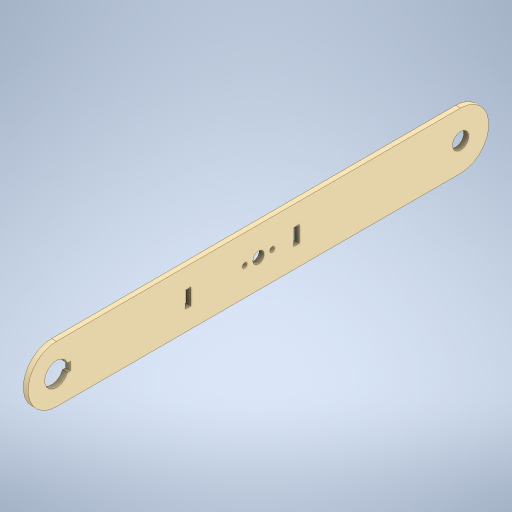
# Autodesk Inventor part: brazo2
Saved by Autodesk Inventor 2024.3 (Build 283343000, 343)
## iProperties
Created: 2024-05-14
Part Number: brazo2
Material: PMMA Plastic
Document SubType Name: Modeling
Designer: USUARIO
Density: 1.188 g/cm^3
Appearance: Beige
Mass: 33.3029 g
Surface Area: 210.325 cm^2
Volume: 28.0327 cm^3
Author: USUARIO
Autodesk Inventor part; units mm, degrees
ref_plane "YZ Plane" through (0, 0, 0) normal (1, 0, 0) x (0, 1, 0)
ref_plane "XZ Plane" through (0, 0, 0) normal (0, 1, 0) x (-1, 0, 0)
ref_plane "XY Plane" through (0, 0, 0) normal (0, 0, 1) x (1, 0, 0)
sketch "Sketch1" plane through (0, 0, 0) normal (1, 0, 0) x (0, 1, 0)
  line L0 (0, 0) -> (0, -250) construction
  circle A0 centre (0, -250) radius 5
  arc A1 (0, -17.5) -> (17.5, 0) centre (0, 0) ccw construction
  arc A2 (0, -232.5) -> (-17.5, -250) centre (0, -250) ccw construction
  line L1 (17.5, 0) -> (17.5, -250)
  line L2 (-17.5, 0) -> (-17.5, -250)
  arc A3 (-17.5, 0) -> (0, -17.5) centre (0, 0) ccw construction
  arc A4 (17.5, 0) -> (-17.5, 0) centre (0, 0) ccw
  arc A5 (17.5, -250) -> (0, -232.5) centre (0, -250) ccw construction
  arc A6 (-17.5, -250) -> (17.5, -250) centre (0, -250) ccw
  line L3 (0, 0) -> (0, -80) construction
  line L4 (0, -80) -> (5, -80) construction
  line L5 (5, -80) -> (5, -83)
  line L6 (5, -83) -> (-5, -83) construction
  line L7 (-5, -83) -> (-5, -80)
  line L8 (-5, -80) -> (0, -80) construction
  line L9 (0, -250) -> (0, -150) construction
  line L10 (0, -150) -> (5, -150) construction
  line L11 (5, -150) -> (5, -147)
  line L12 (5, -147) -> (-5, -147) construction
  line L13 (-5, -147) -> (-5, -150)
  line L14 (0, -150) -> (-5, -150) construction
  line L15 (0, -250) -> (0, -125) construction
  circle A7 centre (0, -125) radius 3.5
  line L16 (0, -125) -> (0, -133.5) construction
  line L17 (0, -125) -> (0, -116.5) construction
  circle A8 centre (0, -116.5) radius 1.5
  circle A9 centre (0, -133.5) radius 1.5
  line L18 (7.5, 0) -> (13.5, 0) construction
  arc A10 (2.5, -6.8053) -> (-2.5, -6.8053) centre (0, 0) ccw
  line L19 (0, -7.25) -> (2.5, -7.25) construction
  line L20 (2.5, -7.25) -> (-2.5, -7.25) construction
  line L21 (-2.5, -7.25) -> (-2.5, -8.75)
  line L22 (-2.5, -8.75) -> (2.5, -8.75)
  line L23 (2.5, -8.75) -> (2.5, -7.25)
  line L24 (2.5, -7.25) -> (2.5, -6.8053)
  line L25 (-2.5, -7.25) -> (-2.5, -6.8053)
  arc A11 (0, -7.25) -> (2.5, -6.8053) centre (0, 0) ccw construction
  arc A12 (-2.5, -6.8053) -> (0, -7.25) centre (0, 0) ccw construction
  line L26 (-5, -80) -> (-5, -79.75)
  line L27 (-5, -79.75) -> (5, -79.75)
  line L28 (5, -79.75) -> (5, -80)
  line L29 (5, -83) -> (5, -83.25)
  line L30 (5, -83.25) -> (-5, -83.25)
  line L31 (-5, -83.25) -> (-5, -83)
  line L32 (5, -150) -> (5, -150.25)
  line L33 (5, -150.25) -> (-5, -150.25)
  line L34 (-5, -150.25) -> (-5, -150)
  line L35 (-5, -147) -> (-5, -146.75)
  line L36 (-5, -146.75) -> (5, -146.75)
  line L37 (5, -146.75) -> (5, -147)
  dimension "d1" = 250
  dimension "d2" = 10
  dimension "d3" = 35
  dimension "d4" = 35
  dimension "d5" = 80
  dimension "d6" = 5
  dimension "d7" = 3
  dimension "d8" = 10
  dimension "d9" = 100
  dimension "d10" = 3
  dimension "d11" = 10
  dimension "d21" = 125
  dimension "d22" = 7
  dimension "d23" = 8.5
  dimension "d24" = 8.5
  dimension "d25" = 3
  dimension "d26" = 3
  dimension "d29" = 14.5
  dimension "d30" = 2.5
  dimension "d31" = 5
  dimension "d32" = 1.5
  dimension "d33" = 0.25
  dimension "d34" = 10
  dimension "d35" = 0.25
  dimension "d36" = 0.25
  dimension "d37" = 10
  dimension "d38" = 0.25
  dimension "d39" = 0.25
  dimension "d40" = 10
  dimension "d41" = 0.25
  dimension "d42" = 0.25
  dimension "d43" = 10
  dimension "d44" = 0.25
  constraints: 76 end point, 18 point on circle, 13 centre point, 13 perpendicular, 13 point on line, 8 coincident, 6 tangent, 6 vertical, 3 parallel, 2 horizontal, 2 midpoint
  measures "d1" distance of L0.start L0.end
  measures "d2" diameter of A0
  measures "d3" diameter of A1
  measures "d4" diameter of A2
  measures "d5" distance of L3.start L3.end
  measures "d6" distance of L3.end L4.end
  measures "d7" distance of L4.end L5.end
  measures "d8" distance of L5.end L6.end
  measures "d9" distance of L9.start L9.end
  measures "d10" distance of L10.end L11.end
  measures "d11" distance of L11.end L12.end
  measures "d21" distance of L9.start L15.end
  measures "d22" diameter of A7
  measures "d23" distance of L16.start L16.end
  measures "d24" distance of L16.start L17.end
  measures "d25" diameter of A8
  measures "d26" diameter of A9
  measures "d29" diameter of A10
  measures "d30" distance of L19.start L19.end
  measures "d31" distance of L22.end L21.end
  measures "d32" distance of L21.end L20.end
  measures "d33" distance of L7.end L26.end
  measures "d34" distance of L26.end L27.end
  measures "d35" distance of L27.end L4.end
  measures "d36" distance of L5.end L29.end
  measures "d37" distance of L29.end L30.end
  measures "d38" distance of L30.end L6.end
  measures "d39" distance of L10.end L32.end
  measures "d40" distance of L32.end L33.end
  measures "d41" distance of L33.end L13.end
  measures "d42" distance of L12.end L35.end
  measures "d43" distance of L35.end L36.end
  measures "d44" distance of L36.end L11.end
extrude "Extrusion1" add sketch "Sketch1" along normal blind 3
body "Solid1"
